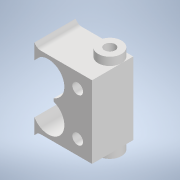
# Autodesk Inventor part: elem
Saved by Autodesk Inventor 2022 (Build 260153000, 153)
## iProperties
Created: 2023-01-17
Part Number: elem
Material: Generic
Document SubType Name: Modeling
Designer: komputer
Density: 1 g/cm^3
Appearance: Default
Author: komputer
Autodesk Inventor part; units mm, degrees
ref_plane "YZ Plane" through (0, 0, 0) normal (1, 0, 0) x (0, 1, 0)
ref_plane "XZ Plane" through (0, 0, 0) normal (0, 1, 0) x (-1, 0, 0)
ref_plane "XY Plane" through (0, 0, 0) normal (0, 0, 1) x (1, 0, 0)
sketch "Sketch1" plane through (0, 0, 0) normal (0, 0, 1) x (1, 0, 0)
  arc A0 (4.4258, -4.7188) -> (3.4446, -4.0254) centre (1.9824, -7.1354) ccw
  arc A1 (4.7101, -4.5588) -> (4.4258, -4.7188) centre (5.9929, -7.1696) ccw
  arc A2 (4.626, -3.3602) -> (4.7101, -4.5588) centre (8.0434, -3.7228) ccw
  arc A3 (5.0611, -3.2311) -> (4.626, -3.3602) centre (5.9929, -7.1696) ccw
  arc A4 (5.6444, -4.2816) -> (5.0611, -3.2311) centre (2.3945, -5.3987) ccw
  arc A5 (5.9699, -4.2608) -> (5.6444, -4.2816) centre (5.9929, -7.1696) ccw
  arc A6 (6.4142, -3.1444) -> (5.9699, -4.2608) centre (9.3358, -4.9538) ccw
  arc A7 (6.8623, -3.2169) -> (6.4142, -3.1444) centre (5.9929, -7.1696) ccw
  arc A8 (6.9319, -4.4164) -> (6.8623, -3.2169) centre (3.5192, -4.0128) ccw
  arc A9 (7.2343, -4.5389) -> (6.9319, -4.4164) centre (5.9929, -7.1696) ccw
  arc A10 (8.119, -3.7258) -> (7.2343, -4.5389) centre (9.9661, -6.6237) ccw
  arc A11 (8.4912, -3.9855) -> (8.119, -3.7258) centre (5.9929, -7.1696) ccw
  arc A12 (8.0335, -5.0965) -> (8.4912, -3.9855) centre (5.1339, -3.2521) ccw
  arc A13 (8.2528, -5.338) -> (8.0335, -5.0965) centre (5.9929, -7.1696) ccw
  arc A14 (9.4026, -4.9894) -> (8.2528, -5.338) centre (9.8095, -8.4017) ccw
  arc A15 (9.6253, -5.3848) -> (9.4026, -4.9894) centre (5.9929, -7.1696) ccw
  arc A16 (8.7309, -6.1872) -> (9.6253, -5.3848) centre (6.9187, -3.2673) ccw
  arc A17 (8.8237, -6.4999) -> (8.7309, -6.1872) centre (5.9929, -7.1696) ccw
  arc A18 (10.0109, -6.6847) -> (8.8237, -6.4999) centre (8.8969, -9.9357) ccw
  arc A19 (10.0399, -7.1376) -> (10.0109, -6.6847) centre (5.9929, -7.1696) ccw
  arc A20 (8.886, -7.4725) -> (10.0399, -7.1376) centre (8.5201, -4.0555) ccw
  arc A21 (8.8339, -7.7945) -> (8.886, -7.4725) centre (5.9929, -7.1696) ccw
  arc A22 (9.8234, -8.4761) -> (8.8339, -7.7945) centre (7.4092, -10.9218) ccw
  arc A23 (9.653, -8.8968) -> (9.8234, -8.4761) centre (5.9929, -7.1696) ccw
  arc A24 (8.4681, -8.6977) -> (9.653, -8.8968) centre (9.621, -5.4604) ccw
  arc A25 (8.2814, -8.9653) -> (8.4681, -8.6977) centre (5.9929, -7.1696) ccw
  arc A26 (8.8772, -10.0087) -> (8.2814, -8.9653) centre (5.6409, -11.1647) ccw
  arc A27 (8.5412, -10.3138) -> (8.8772, -10.0087) centre (5.9929, -7.1696) ccw
  arc A28 (7.5599, -9.6204) -> (8.5412, -10.3138) centre (10.0033, -7.2038) ccw
  arc A29 (7.2757, -9.7804) -> (7.5599, -9.6204) centre (5.9929, -7.1696) ccw
  arc A30 (7.3597, -10.979) -> (7.2757, -9.7804) centre (3.9424, -10.6164) ccw
  arc A31 (6.9246, -11.1081) -> (7.3597, -10.979) centre (5.9929, -7.1696) ccw
  arc A32 (6.3414, -10.0576) -> (6.9246, -11.1081) centre (9.5913, -8.9405) ccw
  arc A33 (6.0158, -10.0784) -> (6.3414, -10.0576) centre (5.9929, -7.1696) ccw
  arc A34 (5.5715, -11.1948) -> (6.0158, -10.0784) centre (2.6499, -9.3853) ccw
  arc A35 (5.1235, -11.1223) -> (5.5715, -11.1948) centre (5.9929, -7.1696) ccw
  arc A36 (5.0538, -9.9228) -> (5.1235, -11.1223) centre (8.4666, -10.3264) ccw
  arc A37 (4.7515, -9.8003) -> (5.0538, -9.9228) centre (5.9929, -7.1696) ccw
  arc A38 (3.8668, -10.6134) -> (4.7515, -9.8003) centre (2.0196, -7.7155) ccw
  arc A39 (3.4946, -10.3537) -> (3.8668, -10.6134) centre (5.9929, -7.1696) ccw
  arc A40 (3.9523, -9.2427) -> (3.4946, -10.3537) centre (6.8519, -11.0871) ccw
  arc A41 (3.733, -9.0012) -> (3.9523, -9.2427) centre (5.9929, -7.1696) ccw
  arc A42 (2.5831, -9.3498) -> (3.733, -9.0012) centre (2.1762, -5.9375) ccw
  arc A43 (2.3605, -8.9544) -> (2.5831, -9.3498) centre (5.9929, -7.1696) ccw
  arc A44 (3.2549, -8.152) -> (2.3605, -8.9544) centre (5.0671, -11.0719) ccw
  arc A45 (3.1621, -7.8393) -> (3.2549, -8.152) centre (5.9929, -7.1696) ccw
  arc A46 (1.9748, -7.6545) -> (3.1621, -7.8393) centre (3.0888, -4.4035) ccw
  arc A47 (1.9458, -7.2016) -> (1.9748, -7.6545) centre (5.9929, -7.1696) ccw
  arc A48 (3.0998, -6.8667) -> (1.9458, -7.2016) centre (3.4656, -10.2837) ccw
  arc A49 (3.1519, -6.5447) -> (3.0998, -6.8667) centre (5.9929, -7.1696) ccw
  arc A50 (2.1623, -5.8631) -> (3.1519, -6.5447) centre (4.5765, -3.4174) ccw
  arc A51 (2.3327, -5.4424) -> (2.1623, -5.8631) centre (5.9929, -7.1696) ccw
  arc A52 (3.5177, -5.6415) -> (2.3327, -5.4424) centre (2.3647, -8.8788) ccw
  arc A53 (3.7043, -5.3739) -> (3.5177, -5.6415) centre (5.9929, -7.1696) ccw
  arc A54 (3.1086, -4.3305) -> (3.7043, -5.3739) centre (6.3448, -3.1745) ccw
  arc A55 (3.4446, -4.0254) -> (3.1086, -4.3305) centre (5.9929, -7.1696) ccw
  circle A56 centre (5.9929, -7.1696) radius 1
  arc A57 (3.4446, -2.1746) -> (4.4258, -1.4812) centre (1.9824, 0.9354) ccw
  arc A58 (3.1086, -1.8695) -> (3.4446, -2.1746) centre (5.9929, 0.9696) ccw
  arc A59 (3.7043, -0.8261) -> (3.1086, -1.8695) centre (6.3448, -3.0255) ccw
  arc A60 (3.5177, -0.5585) -> (3.7043, -0.8261) centre (5.9929, 0.9696) ccw
  arc A61 (2.3327, -0.7576) -> (3.5177, -0.5585) centre (2.3647, 2.6788) ccw
  arc A62 (2.1623, -0.3369) -> (2.3327, -0.7576) centre (5.9929, 0.9696) ccw
  arc A63 (3.1519, 0.3447) -> (2.1623, -0.3369) centre (4.5765, -2.7826) ccw
  arc A64 (3.0998, 0.6667) -> (3.1519, 0.3447) centre (5.9929, 0.9696) ccw
  arc A65 (1.9458, 1.0016) -> (3.0998, 0.6667) centre (3.4656, 4.0837) ccw
  arc A66 (1.9748, 1.4545) -> (1.9458, 1.0016) centre (5.9929, 0.9696) ccw
  arc A67 (3.1621, 1.6393) -> (1.9748, 1.4545) centre (3.0888, -1.7965) ccw
  arc A68 (3.2549, 1.952) -> (3.1621, 1.6393) centre (5.9929, 0.9696) ccw
  arc A69 (2.3605, 2.7544) -> (3.2549, 1.952) centre (5.0671, 4.8719) ccw
  arc A70 (2.5831, 3.1498) -> (2.3605, 2.7544) centre (5.9929, 0.9696) ccw
  arc A71 (3.733, 2.8012) -> (2.5831, 3.1498) centre (2.1762, -0.2625) ccw
  arc A72 (3.9523, 3.0427) -> (3.733, 2.8012) centre (5.9929, 0.9696) ccw
  arc A73 (3.4946, 4.1537) -> (3.9523, 3.0427) centre (6.8519, 4.8871) ccw
  arc A74 (3.8668, 4.4134) -> (3.4946, 4.1537) centre (5.9929, 0.9696) ccw
  arc A75 (4.7515, 3.6003) -> (3.8668, 4.4134) centre (2.0196, 1.5155) ccw
  arc A76 (5.0538, 3.7228) -> (4.7515, 3.6003) centre (5.9929, 0.9696) ccw
  arc A77 (5.1235, 4.9223) -> (5.0538, 3.7228) centre (8.4666, 4.1264) ccw
  arc A78 (5.5715, 4.9948) -> (5.1235, 4.9223) centre (5.9929, 0.9696) ccw
  arc A79 (6.0158, 3.8784) -> (5.5715, 4.9948) centre (2.6499, 3.1853) ccw
  arc A80 (6.3414, 3.8576) -> (6.0158, 3.8784) centre (5.9929, 0.9696) ccw
  arc A81 (6.9246, 4.9081) -> (6.3414, 3.8576) centre (9.5913, 2.7405) ccw
  arc A82 (7.3597, 4.779) -> (6.9246, 4.9081) centre (5.9929, 0.9696) ccw
  arc A83 (7.2757, 3.5804) -> (7.3597, 4.779) centre (3.9424, 4.4164) ccw
  arc A84 (7.5599, 3.4204) -> (7.2757, 3.5804) centre (5.9929, 0.9696) ccw
  arc A85 (8.5412, 4.1138) -> (7.5599, 3.4204) centre (10.0033, 1.0038) ccw
  arc A86 (8.8772, 3.8087) -> (8.5412, 4.1138) centre (5.9929, 0.9696) ccw
  arc A87 (8.2814, 2.7653) -> (8.8772, 3.8087) centre (5.6409, 4.9647) ccw
  arc A88 (8.4681, 2.4977) -> (8.2814, 2.7653) centre (5.9929, 0.9696) ccw
  arc A89 (9.653, 2.6968) -> (8.4681, 2.4977) centre (9.621, -0.7396) ccw
  arc A90 (9.8234, 2.2761) -> (9.653, 2.6968) centre (5.9929, 0.9696) ccw
  arc A91 (8.8339, 1.5945) -> (9.8234, 2.2761) centre (7.4092, 4.7218) ccw
  arc A92 (8.886, 1.2725) -> (8.8339, 1.5945) centre (5.9929, 0.9696) ccw
  arc A93 (10.0399, 0.9376) -> (8.886, 1.2725) centre (8.5201, -2.1445) ccw
  arc A94 (10.0109, 0.4847) -> (10.0399, 0.9376) centre (5.9929, 0.9696) ccw
  arc A95 (8.8237, 0.2999) -> (10.0109, 0.4847) centre (8.8969, 3.7357) ccw
  arc A96 (8.7309, -0.0128) -> (8.8237, 0.2999) centre (5.9929, 0.9696) ccw
  arc A97 (9.6253, -0.8152) -> (8.7309, -0.0128) centre (6.9187, -2.9327) ccw
  arc A98 (9.4026, -1.2106) -> (9.6253, -0.8152) centre (5.9929, 0.9696) ccw
  arc A99 (8.2528, -0.862) -> (9.4026, -1.2106) centre (9.8095, 2.2017) ccw
  arc A100 (8.0335, -1.1035) -> (8.2528, -0.862) centre (5.9929, 0.9696) ccw
  arc A101 (8.4912, -2.2145) -> (8.0335, -1.1035) centre (5.1339, -2.9479) ccw
  arc A102 (8.119, -2.4742) -> (8.4912, -2.2145) centre (5.9929, 0.9696) ccw
  arc A103 (7.2343, -1.6611) -> (8.119, -2.4742) centre (9.9661, 0.4237) ccw
  arc A104 (6.9319, -1.7836) -> (7.2343, -1.6611) centre (5.9929, 0.9696) ccw
  arc A105 (6.8623, -2.9831) -> (6.9319, -1.7836) centre (3.5192, -2.1872) ccw
  arc A106 (6.4142, -3.0556) -> (6.8623, -2.9831) centre (5.9929, 0.9696) ccw
  arc A107 (5.9699, -1.9392) -> (6.4142, -3.0556) centre (9.3358, -1.2462) ccw
  arc A108 (5.6444, -1.9184) -> (5.9699, -1.9392) centre (5.9929, 0.9696) ccw
  arc A109 (5.0611, -2.9689) -> (5.6444, -1.9184) centre (2.3945, -0.8013) ccw
  arc A110 (4.626, -2.8398) -> (5.0611, -2.9689) centre (5.9929, 0.9696) ccw
  arc A111 (4.7101, -1.6412) -> (4.626, -2.8398) centre (8.0434, -2.4772) ccw
  arc A112 (4.4258, -1.4812) -> (4.7101, -1.6412) centre (5.9929, 0.9696) ccw
  circle A113 centre (5.9929, 0.9696) radius 1
  arc A114 (1, -2.8284) -> (-1, -2.8284) centre (0, 0) ccw
  line L0 (1, -3.1) -> (1, -3.3716)
  arc A115 (-1, -3.3716) -> (1, -3.3716) centre (0, -6.2) ccw
  line L1 (1, -2.8284) -> (1, -3.1)
  line L2 (-1, -3.3716) -> (-1, -3.1)
  line L3 (-1, -3.1) -> (-1, -2.8284)
  line L4 (-3.3657, -11.5) -> (14.9623, -11.5)
  line L5 (-3.3657, 5.3) -> (14.9623, 5.3)
  circle A116 centre (0, -6.2) radius 1
  circle A117 centre (0, 0) radius 1
  circle A118 centre (5.9929, -7.1696) radius 3
  circle A119 centre (5.9929, 0.9696) radius 3
  spline S0 degree 3 poles (0.3551, -10.2883) (0.3489, -10.2682) (0.3407, -10.2498) (0.3206, -10.2166) (0.3067, -10.2008) (0.2765, -10.1798) (0.2601, -10.1745) (0.2295, -10.1745) (0.2134, -10.1798) (0.184, -10.2008) (0.1708, -10.2166) (0.1517, -10.2498) (0.144, -10.2682) (0.1381, -10.2883) knots 0 0 0 0 0.148022 0.148022 0.324011 0.324011 0.5 0.5 0.675989 0.675989 0.851978 0.851978 1 1 1 1
  spline S1 degree 3 poles (-0.5985, -10.2883) (-0.6026, -10.2682) (-0.6078, -10.2498) (-0.6208, -10.2166) (-0.6296, -10.2008) (-0.6489, -10.1798) (-0.6592, -10.1745) (-0.6785, -10.1745) (-0.6886, -10.1798) (-0.7068, -10.2008) (-0.715, -10.2166) (-0.7267, -10.2498) (-0.7314, -10.2682) (-0.735, -10.2883) knots 0 0 0 0 0.148022 0.148022 0.324011 0.324011 0.5 0.5 0.675989 0.675989 0.851978 0.851978 1 1 1 1
  spline S2 degree 3 poles (-1.1163, -10.2883) (-1.1178, -10.2682) (-1.1198, -10.2498) (-1.1247, -10.2166) (-1.128, -10.2008) (-1.1349, -10.1798) (-1.1385, -10.1745) (-1.1451, -10.1745) (-1.1484, -10.1798) (-1.1543, -10.2008) (-1.1568, -10.2166) (-1.1604, -10.2498) (-1.1618, -10.2682) (-1.1628, -10.2883) knots 0 0 0 0 0.148022 0.148022 0.324011 0.324011 0.5 0.5 0.675989 0.675989 0.851978 0.851978 1 1 1 1
  line L6 (1.0323, -9.866) -> (-1.9764, -9.866)
  line L7 (-1.3996, -9.866) -> (-1.3996, -11.195)
  line L8 (-1.3996, -11.195) -> (-2.5891, -11.195)
  line L9 (-2.5891, -11.195) -> (-2.5891, -7.7155)
  line L10 (1.0323, -9.866) -> (9.6253, -9.866)
  line L11 (1, -3.1) -> (9.9661, -3.1)
  line L12 (1.0323, 3.666) -> (-1.9764, 3.666)
  line L13 (-1.3996, 3.666) -> (-1.3996, 4.995)
  line L14 (-1.3996, 4.995) -> (-2.5891, 4.995)
  line L15 (-2.5891, 4.995) -> (-2.5891, 1.5155)
  line L16 (1.0323, 3.666) -> (9.6253, 3.666)
  line L17 (5.9929, -7.1696) -> (8.9929, -7.1696)
  line L18 (5.9929, 0.9696) -> (8.9929, 0.9696)
  line L19 (8.9929, -7.1696) -> (8.9929, 0.9696)
  point P0 (7.308, 3.666)
  point P1 (4.9013, 3.666)
  point P2 (4.7001, 3.666)
  point P3 (4.7001, -9.866)
  point P4 (4.9013, -9.866)
  point P5 (7.308, -9.866)
  dimension "d0" = 6
  dimension "d1" = 6
  constraints: 28 end point, 7 symmetric about line, 3 horizontal, 2 coincident, 2 parallel, 2 point on line, 1 perpendicular, 1 point on circle, 1 vertical, 6 other
extrude "Extrusion1" add sketch "Sketch1" against normal blind 10 contours A1 A2 A118 A4 A5 A6 A8 A9 A10 A12 A13 A14 A16 A17 A18 A20 A21 A22 A24 A25 A26 A28 A29 A30 L10 A37 A38 A40 A41 A42 A44 A45 A46 A48 A49 A50 A52 A53 A54 A0 | A0 A118 A2 A1 | A118 A54 A55 A0 | A0 A55 A54 A118 A52 A115 L0 L11 L19 A14 A12 A11 A10 A8 A7 A6 A4 A3 A2 | A2 A3 A4 A118 | A54 A53 A52 A118 | A118 A6 A5 A4 | A118 A50 A115 A52 | A6 A7 A8 A118 | A118 A48 A115 A50 | A50 A49 A48 A118 | A118 A10 A9 A8 | A118 A46 A115 A48 | A10 A11 A12 A118 | L1 A114 A61 A119 A59 A58 A57 A111 A110 A109 A107 A106 A105 A103 A102 A101 A99 L19 L11 | A118 A44 A43 A42 A40 L10 L6 L7 L8 L9 A115 A46 | A46 A45 A44 A118 | A118 A14 A13 A12 | A118 A42 A43 A44 | A14 L19 A16 A118 | A114 A63 A119 A61 | A99 A119 A97 L19 | A42 A41 A40 A118 | A118 A18 A17 A16 | A16 L19 A18 A118 | A119 A63 A64 A65 A67 A68 A69 A71 A72 A73 L16 A75 A76 A83 A84 A85 A87 A88 A89 A91 A92 A93 A95 A96 A97 A99 A100 A101 A103 A104 A105 A107 A108 A109 A111 A112 A57 A59 A60 A61 | A61 A60 A59 A119 | A114 A65 A119 A63 | A119 A101 A100 A99 | A97 A119 A95 L19 | A118 L10 A40 | A18 L19 A118 | A119 A65 A64 A63 | A119 A57 A58 A59 | A114 A67 A119 A65 | A101 A102 A103 A119 | A97 A96 A95 A119 | A95 A119 L19 | A57 A112 A111 A119 | A114 L15 L14 L13 L12 L16 A73 A119 A71 A70 A69 A67 | A119 A105 A104 A103 | A118 A22 A21 A20 | A119 A69 A68 A67 | A119 A109 A110 A111 | A105 A106 A107 A119 | A93 A92 A91 A119 | A69 A70 A71 A119 | A109 A108 A107 A119 | A30 A29 A28 A118 L10 | A118 A26 A25 A24 | A119 A73 A72 A71 | A89 A88 A87 A119 | A73 L16 A119 | A85 A84 A83 L16 A119
sketch "Sketch2" plane through (0, 0, -10) normal (0, 0, -1) x (-1, 0, 0)
  arc A0 (-7.308, 3.666) -> (-8.9929, 0.9696) centre (-5.9929, 0.9696) ccw projected
  line L0 (-8.9929, 0.9696) -> (-8.9929, -7.1696) projected
  arc A1 (-8.9929, -7.1696) -> (-7.308, -9.866) centre (-5.9929, -7.1696) ccw projected
  line L1 (-7.308, -9.866) -> (-4.9013, -9.866) projected
  arc A2 (-4.9013, -9.866) -> (-4.7515, -9.8003) centre (-5.9929, -7.1696) ccw projected
  arc A3 (-4.7515, -9.8003) -> (-4.7001, -9.866) centre (-2.0196, -7.7155) ccw projected
  line L2 (-4.7001, -9.866) -> (1.3996, -9.866) projected
  line L3 (1.3996, -9.866) -> (1.3996, -11.195) projected
  line L4 (1.3996, -11.195) -> (2.5891, -11.195) projected
  line L5 (2.5891, -11.195) -> (2.5891, -7.7155) projected
  arc A4 (-1, -3.3716) -> (2.5891, -7.7155) centre (0, -6.2) ccw projected
  line L6 (-1, -3.3716) -> (-1, -2.8284) projected
  arc A5 (2.5891, 1.5155) -> (-1, -2.8284) centre (0, 0) ccw projected
  line L7 (2.5891, 1.5155) -> (2.5891, 4.995) projected
  line L8 (2.5891, 4.995) -> (1.3996, 4.995) projected
  line L9 (1.3996, 4.995) -> (1.3996, 3.666) projected
  line L10 (1.3996, 3.666) -> (-4.7001, 3.666) projected
  arc A6 (-4.7001, 3.666) -> (-4.7515, 3.6003) centre (-2.0196, 1.5155) ccw projected
  arc A7 (-4.7515, 3.6003) -> (-4.9013, 3.666) centre (-5.9929, 0.9696) ccw projected
  line L11 (-4.9013, 3.666) -> (-7.308, 3.666) projected
  circle A8 centre (-5.9929, -7.1696) radius 1 projected
  circle A9 centre (-5.9929, 0.9696) radius 1 projected
  arc A10 (-4.7515, -9.8003) -> (-4.7001, -9.866) centre (-2.0196, -7.7155) ccw projected
  line L12 (-4.9013, -9.866) -> (-4.7001, -9.866)
  line L13 (-4.9013, 3.666) -> (-4.7001, 3.666)
  point P0 (0, 0)
  constraints: 4 end point, 1 horizontal
extrude "Extrusion2" add sketch "Sketch2" against normal blind 10 contours L13 A6 A7 | A2 A3 L12
sketch "Sketch3" plane through (-1.3996, -9.866, 0) normal (0, -1, 0) x (1, 0, 0)
  line L0 (8.3925, -10) -> (6.3925, -10) projected
  line L1 (6.3925, 0) -> (8.3925, 0) projected
  circle A0 centre (7.1979, -5.5076) radius 1 projected
  line L2 (8.3925, -10) -> (6.3925, -10) projected
  line L3 (7.3925, -10) -> (7.3925, 0)
  line L4 (0, 0) -> (8.7076, 0) projected
  line L5 (7.1979, -5.5076) -> (7.3925, -5.5076)
  circle A1 centre (7.3925, -5.5076) radius 1
  point P0 (1.3996, 0)
  dimension "d6" = 2
  constraints: 4 end point, 2 perpendicular, 2 point on line, 1 centre point, 1 coincident, 1 midpoint
  measures "d6" diameter of A1
extrude "Extrusion3" cut sketch "Sketch3" against normal through all contours A0 L3 | A0 L3 A1 | L3 A0 A1 | A0 A1 L3 | L3 A1 A0
sketch "Sketch4" plane through (-1.3996, 3.666, 0) normal (0, 1, 0) x (1, 0, 0)
  circle A0 centre (7.3925, 5.5076) radius 1 projected
  circle A1 centre (7.3925, 5.5076) radius 2.1832
  point P0 (1.3996, 0)
  constraints: 1 centre point, 1 coincident
extrude "Extrusion4" add sketch "Sketch4" along normal blind 1.5
extrude "Extrusion5" add sketch "Sketch4" against normal blind 1
sketch "Sketch5" plane through (5.9929, 5.166, -5.5076) normal (0, 1, 0) x (1, 0, 0)
  arc A0 (1, 0) -> (-1, 0) centre (0, 0) ccw projected
  circle A1 centre (0, 0) radius 2.1832 projected
  circle A2 centre (0, 0) radius 1 projected
  point P0 (-5.9929, -5.5076)
  point P1 (-1, 0)
extrude "Extrusion6" add sketch "Sketch5" against normal blind 16.532
sketch "Sketch6" plane through (0, 0, -10) normal (0, 0, -1) x (-1, 0, 0)
  spline S0 degree 5 poles (-6.9929, -7.1696) (-6.9929, -7.0677) (-6.9799, -6.966) (-6.954, -6.8663) (-6.9155, -6.7703) (-6.7874, -6.542) (-6.6812, -6.4173) (-6.5484, -6.3108) (-6.3865, -6.2329) (-6.0378, -6.155) (-5.8509, -6.1533) (-5.6691, -6.1993) (-5.5139, -6.2765) (-5.2309, -6.494) (-5.1134, -6.6421) (-5.0334, -6.8107) (-4.9929, -6.9899) (-4.9929, -7.2715) (-5.0058, -7.3732) (-5.0317, -7.4729) (-5.0702, -7.5689) (-5.1983, -7.7971) (-5.3046, -7.9219) (-5.4373, -8.0284) (-5.5993, -8.1063) (-5.948, -8.1842) (-6.1348, -8.1859) (-6.3167, -8.1399) (-6.4719, -8.0627) (-6.7547, -7.8452) (-6.8721, -7.6969) (-6.9524, -7.529) (-6.9929, -7.3494) (-6.9929, -7.1696) knots 0 0 0 0 0 0 0.085801 0.085801 0.085801 0.085801 0.217494 0.217494 0.217494 0.217494 0.347535 0.347535 0.347535 0.347535 0.499266 0.499266 0.499266 0.499266 0.585331 0.585331 0.585331 0.585331 0.717428 0.717428 0.717428 0.717428 0.847868 0.847868 0.847868 0.847868 1 1 1 1 1 1 projected
  spline S1 degree 5 poles (-6.9929, 0.9696) (-6.9929, 1.0715) (-6.9799, 1.1732) (-6.954, 1.2729) (-6.9155, 1.3689) (-6.7874, 1.5971) (-6.6812, 1.7219) (-6.5484, 1.8284) (-6.3865, 1.9063) (-6.0378, 1.9842) (-5.8509, 1.9859) (-5.6691, 1.9399) (-5.5139, 1.8627) (-5.2309, 1.6452) (-5.1134, 1.4971) (-5.0334, 1.3285) (-4.9929, 1.1493) (-4.9929, 0.8677) (-5.0058, 0.766) (-5.0317, 0.6663) (-5.0702, 0.5703) (-5.1983, 0.342) (-5.3046, 0.2173) (-5.4373, 0.1108) (-5.5993, 0.0329) (-5.948, -0.045) (-6.1348, -0.0467) (-6.3167, -0.0007) (-6.4719, 0.0765) (-6.7547, 0.294) (-6.8721, 0.4423) (-6.9524, 0.6102) (-6.9929, 0.7898) (-6.9929, 0.9696) knots 0 0 0 0 0 0 0.085801 0.085801 0.085801 0.085801 0.217494 0.217494 0.217494 0.217494 0.347535 0.347535 0.347535 0.347535 0.499266 0.499266 0.499266 0.499266 0.585331 0.585331 0.585331 0.585331 0.717428 0.717428 0.717428 0.717428 0.847868 0.847868 0.847868 0.847868 1 1 1 1 1 1 projected
  point P0 (0, 0)
  constraints: 2 other
extrude "Extrusion7" cut sketch "Sketch6" against normal through all
sketch "Sketch7" plane through (0, 0, 0) normal (0, 0, 1) x (1, 0, 0)
  arc A0 (8.9929, 0.9696) -> (7.308, 3.666) centre (5.9929, 0.9696) ccw projected
  line L0 (7.308, 3.666) -> (-1.3996, 3.666) projected
  line L1 (-1.3996, 3.666) -> (-1.3996, 4.995) projected
  line L2 (-1.3996, 4.995) -> (-2.5891, 4.995) projected
  line L3 (-2.5891, 4.995) -> (-2.5891, 1.5155) projected
  arc A1 (1, -2.8284) -> (-2.5891, 1.5155) centre (0, 0) ccw projected
  line L4 (1, -2.8284) -> (1, -3.3716) projected
  arc A2 (-2.5891, -7.7155) -> (1, -3.3716) centre (0, -6.2) ccw projected
  line L5 (-2.5891, -7.7155) -> (-2.5891, -11.195) projected
  line L6 (-2.5891, -11.195) -> (-1.3996, -11.195) projected
  line L7 (-1.3996, -11.195) -> (-1.3996, -9.866) projected
  line L8 (-1.3996, -9.866) -> (7.308, -9.866) projected
  arc A3 (7.308, -9.866) -> (8.9929, -7.1696) centre (5.9929, -7.1696) ccw projected
  line L9 (8.9929, -7.1696) -> (8.9929, 0.9696) projected
  circle A4 centre (5.9929, -7.1696) radius 1 projected
  circle A5 centre (5.9929, 0.9696) radius 1 projected
  line L10 (4.9929, 5.166) -> (6.9929, 5.166) projected
  line L11 (7.308, 3.666) -> (-1.3996, 3.666) projected
  arc A6 (8.9929, 0.9696) -> (7.308, 3.666) centre (5.9929, 0.9696) ccw projected
  line L12 (7.308, 3.666) -> (8.9929, 3.666)
  line L13 (8.9929, 3.666) -> (8.9929, 0.9696)
  line L14 (8.9929, 0.9696) -> (7.308, 0.9696)
  line L15 (7.308, 0.9696) -> (7.308, 3.666)
  line L16 (7.308, -9.866) -> (8.9929, -9.866)
  line L17 (8.9929, -9.866) -> (8.9929, -7.1696)
  line L18 (8.9929, -7.1696) -> (7.308, -7.1696)
  line L19 (7.308, -7.1696) -> (7.308, -9.866)
  line L20 (8.9929, -9.866) -> (10.4929, -9.866)
  line L21 (10.4929, -9.866) -> (10.4929, 3.666)
  line L22 (10.4929, 3.666) -> (8.9929, 3.666)
  line L23 (8.9929, 3.666) -> (8.9929, -9.866)
  point P0 (0, 0)
  point P1 (8.9929, -7.1696)
  dimension "d17" = 1.5
  constraints: 24 end point, 6 parallel, 3 horizontal, 3 perpendicular, 3 point on circle, 2 point on line
  measures "d17" distance of L22.end L21.end
extrude "Extrusion8" add sketch "Sketch7" against normal up to surface (10 mm away) contours L13 L22 L21 L20 L17 L9 | A0 L12 L13 | L17 L16 A3 | A3 L19 L18
sketch "Sketch8" plane through (0, 0, -10) normal (0, 0, -1) x (-1, 0, 0)
  circle A0 centre (-5.9929, 0.9696) radius 1 projected
  circle A1 centre (-5.9929, -7.1696) radius 1 projected
  line L0 (-10.4929, -9.866) -> (1.3996, -9.866) projected
  line L1 (1.3996, -9.866) -> (1.3996, -11.195) projected
  line L2 (1.3996, -11.195) -> (2.5891, -11.195) projected
  line L3 (2.5891, -11.195) -> (2.5891, -7.7155) projected
  arc A2 (-1, -3.3716) -> (2.5891, -7.7155) centre (0, -6.2) ccw projected
  line L4 (-1, -3.3716) -> (-1, -2.8284) projected
  arc A3 (2.5891, 1.5155) -> (-1, -2.8284) centre (0, 0) ccw projected
  line L5 (2.5891, 1.5155) -> (2.5891, 4.995) projected
  line L6 (2.5891, 4.995) -> (1.3996, 4.995) projected
  line L7 (1.3996, 4.995) -> (1.3996, 3.666) projected
  line L8 (1.3996, 3.666) -> (-10.4929, 3.666) projected
  line L9 (-10.4929, 3.666) -> (-10.4929, -9.866) projected
  line L10 (-5.9929, -7.1696) -> (-5.4929, -7.1696)
  circle A4 centre (-5.4929, -7.1696) radius 1
  circle A5 centre (-5.4929, 0.9696) radius 1
  point P0 (0, 0)
  point P1 (-5.7429, 0.0014)
  point P2 (-5.7429, 1.9378)
  point P3 (-5.7429, -8.1378)
  point P4 (-5.7429, -6.2014)
  dimension "d20" = 0.5
  constraints: 2 centre point, 2 end point, 1 coincident, 1 horizontal
  measures "d20" distance of L10.start L10.end
extrude "Extrusion9" add sketch "Sketch8" against normal up to surface (10 mm away) contours A5 A0 | A4 A1 picked at (-6.8189, 1.0094) picked at (-6.8189, -7.1298)
extrude "Extrusion10" cut sketch "Sketch8" against normal through all contours A0 A5 | A1 A4 picked at (-4.6682, 0.8943) picked at (-4.6682, -7.2449)
sketch "Sketch9" plane through (0, 0, -10) normal (0, 0, -1) x (-1, 0, 0)
  circle A0 centre (-5.4929, -7.1696) radius 1 projected
  circle A1 centre (-5.4929, 0.9696) radius 1 projected
  line L0 (-10.4929, -9.866) -> (1.3996, -9.866) projected
  line L1 (1.3996, -9.866) -> (1.3996, -11.195) projected
  line L2 (1.3996, -11.195) -> (2.5891, -11.195) projected
  line L3 (2.5891, -11.195) -> (2.5891, -7.7155) projected
  arc A2 (-1, -3.3716) -> (2.5891, -7.7155) centre (0, -6.2) ccw projected
  line L4 (-1, -3.3716) -> (-1, -2.8284) projected
  arc A3 (2.5891, 1.5155) -> (-1, -2.8284) centre (0, 0) ccw projected
  line L5 (2.5891, 1.5155) -> (2.5891, 4.995) projected
  line L6 (2.5891, 4.995) -> (1.3996, 4.995) projected
  line L7 (1.3996, 4.995) -> (1.3996, 3.666) projected
  line L8 (1.3996, 3.666) -> (-10.4929, 3.666) projected
  line L9 (-10.4929, 3.666) -> (-10.4929, -9.866) projected
  line L10 (1.3996, -11.195) -> (2.5891, -11.195) projected
  line L11 (1.3996, -9.866) -> (1.3996, -11.195) projected
  circle A4 centre (1.3996, -11.195) radius 1.329
  line L12 (1.3996, 4.995) -> (1.3996, 3.666) projected
  circle A5 centre (1.3996, 4.995) radius 1.329
  point P0 (0, 0)
  constraints: 2 coincident, 2 vertical alignment, 4 other
extrude "Extrusion11" cut sketch "Sketch9" against normal blind 10 contours A4 L3 L2 L1 | L1 L2 L3 A4 | A5 L5 L6 L7 | L7 L6 L5 A5
sketch "Sketch10" plane through (0, 0, -10) normal (0, 0, -1) x (-1, 0, 0)
  point P0 (0, 0)
sketch "Sketch11" plane through (0, 0, -10) normal (0, 0, -1) x (-1, 0, 0)
  arc A0 (1.3996, 3.666) -> (2.5891, 4.4022) centre (1.3996, 4.995) ccw projected
  line L0 (1.3996, 3.666) -> (-10.4929, 3.666) projected
  line L1 (-10.4929, 3.666) -> (-10.4929, -9.866) projected
  line L2 (-10.4929, -9.866) -> (1.3996, -9.866) projected
  arc A1 (2.5891, -10.6022) -> (1.3996, -9.866) centre (1.3996, -11.195) ccw projected
  line L3 (2.5891, -10.6022) -> (2.5891, -7.7155) projected
  arc A2 (-1, -3.3716) -> (2.5891, -7.7155) centre (0, -6.2) ccw projected
  line L4 (-1, -3.3716) -> (-1, -2.8284) projected
  arc A3 (2.5891, 1.5155) -> (-1, -2.8284) centre (0, 0) ccw projected
  line L5 (2.5891, 1.5155) -> (2.5891, 4.4022) projected
  circle A4 centre (-5.4929, -7.1696) radius 1 projected
  circle A5 centre (-5.4929, 0.9696) radius 1 projected
  line L6 (-8.1761, 3.666) -> (-8.1761, 5.166) projected
  line L7 (-8.1761, -9.866) -> (-8.1761, -11.366) projected
  line L8 (-10.4929, 3.666) -> (-8.1761, 3.666)
  line L9 (-8.1761, 3.666) -> (-8.1761, -9.866)
  line L10 (-8.1761, -9.866) -> (-10.4929, -9.866)
  line L11 (-10.4929, -9.866) -> (-10.4929, 3.666)
  point P0 (0, 0)
  constraints: 8 end point, 2 parallel, 1 horizontal, 1 perpendicular
extrude "Extrusion12" cut sketch "Sketch11" against normal through all contours L9 L2 L1 L0
sketch "Sketch12" plane through (0, 0, -10) normal (0, 0, -1) x (-1, 0, 0)
  circle A0 centre (-5.4929, 0.9696) radius 1 projected
  circle A1 centre (-5.4929, -7.1696) radius 1 projected
  line L0 (-8.1761, 3.666) -> (-8.1761, -9.866) projected
  line L1 (-8.1761, -9.866) -> (1.3996, -9.866) projected
  arc A2 (2.5891, -10.6022) -> (1.3996, -9.866) centre (1.3996, -11.195) ccw projected
  line L2 (2.5891, -10.6022) -> (2.5891, -7.7155) projected
  arc A3 (-1, -3.3716) -> (2.5891, -7.7155) centre (0, -6.2) ccw projected
  line L3 (-1, -3.3716) -> (-1, -2.8284) projected
  arc A4 (2.5891, 1.5155) -> (-1, -2.8284) centre (0, 0) ccw projected
  line L4 (2.5891, 1.5155) -> (2.5891, 4.4022) projected
  arc A5 (1.3996, 3.666) -> (2.5891, 4.4022) centre (1.3996, 4.995) ccw projected
  line L5 (1.3996, 3.666) -> (-8.1761, 3.666) projected
  point P0 (0, 0)
extrude "Extrusion13" cut sketch "Sketch12" against normal blind 2.3
body "Solid1"
